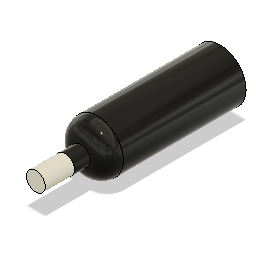
air tank v1 (Autodesk Fusion 360 design; units mm, degrees)
Autodesk Fusion 360 part; units mm, degrees
sketch "Sketch1" plane through (0, 0, 0) normal (0, 0, 1) x (1, 0, 0)
  circle A0 centre (0, 0) radius 41.5
  dimension "d1" = 83
  measures "d1" diameter of A0
extrude "Extrude1" add sketch "Sketch1" along normal blind 223 makes body 1
sketch "Sketch2" plane through (0, 0, 223) normal (0, 0, 1) x (1, 0, 0)
  circle A0 centre (0, 0) radius 41.5
  circle A1 centre (0, 0) radius 15
  circle A2 centre (0, 0) radius 15
  dimension "d4" = 30
  measures "d4" diameter of A1
extrude "Extrude2" add sketch "Sketch2" along normal blind 25 contours A1 A2 bodies 1
fillet "Fillet1" radius 26.5 1 edges at (-38.6916, -15.007, 223) on bodies 1
sketch "Sketch3" plane through (0, 0, 248) normal (0, 0, 1) x (1, 0, 0)
  circle A0 centre (0, 0) radius 15
  circle A1 centre (0, 0) radius 15
extrude "Extrude3" add sketch "Sketch3" along normal blind 47 separate body makes body 2
